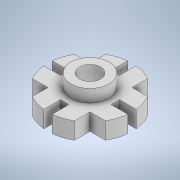
# Autodesk Inventor part: IndexingGuide
Saved by Autodesk Inventor 2022.2 (Build 262287030, 287C)
## iProperties
Created: 2023-02-24
Part Number: IndexingGuide
Material: Generic
Document SubType Name: Modeling
Designer: jak27277
Density: 1 g/cm^3
Appearance: Default
Author: jak27277
Autodesk Inventor part; units mm, degrees
ref_plane "YZ Plane" through (0, 0, 0) normal (1, 0, 0) x (0, 1, 0)
ref_plane "XZ Plane" through (0, 0, 0) normal (0, 1, 0) x (-1, 0, 0)
ref_plane "XY Plane" through (0, 0, 0) normal (0, 0, 1) x (1, 0, 0)
sketch "Sketch1" plane through (0, 0, 0) normal (0, 1, 0) x (-1, 0, 0)
  circle A0 centre (0, 0) radius 63.5
  dimension "d0" = 127
  constraints: 1 centre point, 1 coincident
  measures "d0" diameter of A0
extrude "Extrusion1" add sketch "Sketch1" along normal blind 25.4
sketch "Sketch2" plane through (0, 25.4, 0) normal (0, 1, 0) x (1, 0, 0)
  circle A0 centre (0, 0) radius 28.575
  dimension "d3" = 57.15
  constraints: 1 centre point, 1 coincident
  measures "d3" diameter of A0
extrude "Extrusion2" add sketch "Sketch2" along normal blind 19.05
sketch "Sketch3" plane through (0, 44.45, 0) normal (0, 1, 0) x (1, 0, 0)
  point P0 (0, 0)
  point P1 (0, 0)
  constraints: 1 coincident
hole "Hole1" at (0, 44.45, 0) direction (0, -1, 0) diameter 31.75 end through all
sketch "Sketch4" plane through (0, 25.4, 0) normal (0, 1, 0) x (1, 0, 0)
  line L0 (0, 0) -> (0, 86.5817)
  line L1 (-6.35, 63.5) -> (6.35, 63.5)
  line L2 (6.35, 63.5) -> (6.35, 38.1)
  line L3 (6.35, 38.1) -> (-6.35, 38.1)
  line L4 (-6.35, 38.1) -> (-6.35, 63.5)
  circle A0 centre (0, 0) radius 63.5 projected
  line L5 (0, 0) -> (96.5771, 0)
  circle A1 centre (0, 0) radius 63.5 projected
  line L6 (31.75, 54.9926) -> (31.75, 31.75)
  line L7 (31.75, 31.75) -> (54.9926, 31.75)
  line L8 (-38.1, -6.35) -> (-63.5, -6.35)
  line L9 (-63.5, -6.35) -> (-63.5, 6.35)
  line L10 (-38.1, 6.35) -> (-38.1, -6.35)
  line L11 (-63.5, 6.35) -> (-38.1, 6.35)
  line L12 (-54.9926, 31.75) -> (-31.75, 31.75)
  line L13 (-31.75, 31.75) -> (-31.75, 54.9926)
  line L14 (6.35, -38.1) -> (6.35, -63.5)
  line L15 (6.35, -63.5) -> (-6.35, -63.5)
  line L16 (-6.35, -38.1) -> (6.35, -38.1)
  line L17 (-6.35, -63.5) -> (-6.35, -38.1)
  line L18 (-31.75, -54.9926) -> (-31.75, -31.75)
  line L19 (-31.75, -31.75) -> (-54.9926, -31.75)
  line L20 (38.1, 6.35) -> (63.5, 6.35)
  line L21 (63.5, 6.35) -> (63.5, -6.35)
  line L22 (38.1, -6.35) -> (38.1, 6.35)
  line L23 (63.5, -6.35) -> (38.1, -6.35)
  line L24 (54.9926, -31.75) -> (31.75, -31.75)
  line L25 (31.75, -31.75) -> (31.75, -54.9926)
  point P0 (0, 43.2908)
  point P1 (-63.1817, 6.35)
  point P2 (-63.1817, -6.35)
  point P3 (-6.35, -63.1817)
  point P4 (6.35, -63.1817)
  point P5 (63.1817, -6.35)
  point P6 (63.1817, 6.35)
  point P7 (6.35, 63.1817)
  point P8 (-6.35, 63.1817)
  dimension "d13" = 12.7
  dimension "d14" = 76.2
  dimension "d15" = 63.5
  dimension "d16" = 63.5
  dimension "d19" = 360
  constraints: 52 end point, 3 horizontal, 2 parallel, 2 perpendicular, 2 vertical, 1 midpoint, 58 other
  measures "d13" distance of L2.end L3.end
  measures "d14" diameter of L3 L5
  measures "d15" diameter of L7 L5
  measures "d16" diameter of L6 point (0, 43.291)
extrude "Extrusion3" cut sketch "Sketch4" against normal through all contours L3 L4 A0 L0 | L0 A0 L2 L3 | L22 L20 A0 L5 | L5 A0 L23 L22 | A0 L7 L6 | L13 L12 A0 | A0 L25 L24 | L11 L10 L8 A0 | A0 L17 L16 L14 | L19 L18 A0
body "Solid1"
